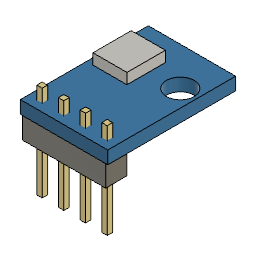
Case_Temperature__Humidity_Sensor (Autodesk Fusion 360 archive; units mm, degrees)
design "AHT10"
part number: 2026-08-29-19-32-47-805
Autodesk Fusion 360 part; units mm, degrees
sketch "Sketch1" plane through (0, 0, 0) normal (0, 0, 1) x (1, 0, 0)
  line L0 (-5.125, 7.5) -> (5.125, 7.5)
  line L1 (5.125, 7.5) -> (5.125, -7.5)
  line L2 (5.125, -7.5) -> (-5.125, -7.5)
  line L3 (-5.125, -7.5) -> (-5.125, 7.5)
  circle A0 centre (3.125, 3) radius 1.625
  line L4 (-4.375, 4.75) -> (-0.375, 4.75)
  line L5 (-0.375, 4.75) -> (-0.375, 0.25)
  line L6 (-0.375, 0.25) -> (-4.375, 0.25)
  line L7 (-4.375, 0.25) -> (-4.375, 4.75)
  line L8 (-1.27, -6.25) -> (1.27, -6.25) construction
  line L9 (-1.59, -5.93) -> (-0.95, -5.93)
  line L10 (-0.95, -5.93) -> (-0.95, -6.57)
  line L11 (-0.95, -6.57) -> (-1.59, -6.57)
  line L12 (-1.59, -6.57) -> (-1.59, -5.93)
  line L13 (0.95, -5.93) -> (1.59, -5.93)
  line L14 (1.59, -5.93) -> (1.59, -6.57)
  line L15 (1.59, -6.57) -> (0.95, -6.57)
  line L16 (0.95, -6.57) -> (0.95, -5.93)
  line L17 (-4.875, -5) -> (4.875, -5)
  line L18 (4.875, -5) -> (4.875, -7.5)
  line L19 (4.875, -7.5) -> (-4.875, -7.5)
  line L20 (-4.875, -7.5) -> (-4.875, -5)
  line L21 (-4.13, -5.93) -> (-3.49, -5.93)
  line L22 (-3.49, -5.93) -> (-3.49, -6.57)
  line L23 (-3.49, -6.57) -> (-4.13, -6.57)
  line L24 (-4.13, -6.57) -> (-4.13, -5.93)
  line L25 (3.49, -5.93) -> (4.13, -5.93)
  line L26 (4.13, -5.93) -> (4.13, -6.57)
  line L27 (4.13, -6.57) -> (3.49, -6.57)
  line L28 (3.49, -6.57) -> (3.49, -5.93)
  point P0 (0, 7.5)
  point P1 (5.125, 0)
  point P2 (1.27, -5.93)
  point P3 (1.59, -6.25)
  point P4 (-1.27, -5.93)
  point P5 (-1.59, -6.25)
  point P6 (0, -6.25)
  point P7 (4.875, -6.25)
  point P8 (0, -5)
  dimension "d1" = 10.25
  dimension "d2" = 15
  dimension "d3" = 2
  dimension "d4" = 4.5
  dimension "d5" = 3.25
  dimension "d6" = 4
  dimension "d7" = 4.5
  dimension "d8" = 4.75
  dimension "d9" = 7.25
  dimension "d10" = 0.64
  dimension "d11" = 2.54
  dimension "d12" = 2.5
  dimension "d13" = 9.75
  dimension "d14" = 1.9
  dimension "d15" = 1.9
  dimension "d16" = 1.9
  constraint horizontal L0
  constraint vertical L1
  constraint horizontal L2
  constraint vertical L3
  constraint midpoint L0 P0
  constraint midpoint L1 P1
  constraint vertical origin P0
  constraint horizontal origin P1
  constraint horizontal L4
  constraint vertical L5
  constraint horizontal L6
  constraint vertical L7
  constraint parallel L2 L8
  constraint horizontal L9
  constraint vertical L10
  constraint horizontal L11
  constraint vertical L12
  constraint horizontal L13
  constraint vertical L14
  constraint horizontal L15
  constraint vertical L16
  constraint midpoint L13 P2
  constraint midpoint L14 P3
  constraint midpoint L9 P4
  constraint midpoint L12 P5
  constraint horizontal L8.start P5
  constraint vertical L8.start P4
  constraint vertical L8.end P2
  constraint horizontal L8.end P3
  constraint equal L13 L14
  constraint equal L10 L13
  constraint equal L9 L13
  constraint midpoint L8 P6
  constraint vertical origin P6
  constraint horizontal L17
  constraint vertical L18
  constraint horizontal L19
  constraint vertical L20
  constraint midpoint L18 P7
  constraint horizontal P3 P7
  constraint midpoint L17 P8
  constraint vertical origin P8
  constraint collinear L2 L19
  constraint horizontal L21
  constraint vertical L22
  constraint horizontal L23
  constraint vertical L24
  constraint horizontal L25
  constraint vertical L26
  constraint horizontal L27
  constraint vertical L28
  constraint equal L25 L26
  constraint equal L21 L22
  constraint equal L12 L22
  constraint equal L14 L28
  constraint collinear L9 L21
  constraint collinear L13 L25
  measures "d1" distance of L0.start L0.end
  measures "d2" distance of L0.start L2.end
  measures "d3" distance of L1 A0.centre
  measures "d4" distance of L0 A0.centre
  measures "d5" diameter of A0
  measures "d6" distance of L4.start L4.end
  measures "d7" distance of L4.start L6.end
  measures "d8" distance of L3 L5
  measures "d9" distance of L0 L6
  measures "d10" distance of L13.start L13.end
  measures "d11" distance of L8.start L8.end
  measures "d12" distance of L17.end L18.end
  measures "d13" distance of L17.start L17.end
  measures "d14" distance of L10 L16
  measures "d15" distance of L14 L28
  measures "d16" distance of L9.start L21.end
extrude "Extrude1" add sketch "Sketch1" against normal blind 1.5 contours L0 L1 L2 L3 L17 L18 L20 | L2 L17 L18 L19 L20 | L4 L5 L6 L7 | L9 L10 L11 L12 | L13 L14 L15 L16 | L21 L22 L23 L24 | L25 L26 L27 L28 makes body 1
extrude "Extrude2" add sketch "Sketch1" along normal blind 1.25 separate body contours L4 L5 L6 L7 makes body 2
extrude "Extrude3" add sketch "Sketch1" against normal blind 11.15 from surface at 1.5 separate body contours L9 L10 L11 L12 | L13 L14 L15 L16 | L21 L22 L23 L24 | L25 L26 L27 L28 makes body 3 at (-3.9167, -5.93, -5.9333) makes body 4 at (1.59, -6.1433, -5.9333) makes body 5 at (-0.95, -6.1433, -5.9333) makes body 6 at (3.7033, -5.93, -2.2167)
extrude "Extrude4" add sketch "Sketch1" against normal blind 2.5 from surface at -1.5 separate body contours L2 L17 L18 L19 L20 makes body 7
equation "d15 = d14"
equation "d16 = d14"
